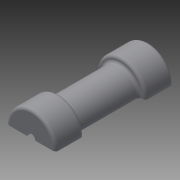
# Autodesk Inventor part: resistor
Saved by Autodesk Inventor 2015 (Build 190159000, 159)
## iProperties
Created: 2014-07-26
Part Number: resistor
Material: Generic
Document SubType Name: Modeling
Designer: dan
Density: 1 g/cm^3
Appearance: Default
Author: dan
Autodesk Inventor part; units mm, degrees
ref_plane "YZ Plane" through (0, 0, 0) normal (1, 0, 0) x (0, 1, 0)
ref_plane "XZ Plane" through (0, 0, 0) normal (0, 1, 0) x (-1, 0, 0)
ref_plane "XY Plane" through (0, 0, 0) normal (0, 0, 1) x (1, 0, 0)
sketch "Sketch1" plane through (0, 0, 0) normal (0, 1, 0) x (-1, 0, 0)
  arc A0 (379.6785, 346.6237) -> (348.5368, 347.4661) centre (364.5795, 364.4873) ccw
  circle A1 centre (364.5795, 364.4873) radius 10.6303
  line L0 (0, 0) -> (12.7, 0)
  line L1 (12.7, 0) -> (12.7, -14.605)
  line L2 (12.7, -14.605) -> (0, -14.605)
  line L3 (0, -14.605) -> (0, 0)
  line L4 (0, -14.605) -> (9.525, -14.605)
  line L5 (9.525, -14.605) -> (9.525, -46.355)
  line L6 (9.525, -46.355) -> (0, -46.355)
  line L7 (0, -46.355) -> (0, -14.605)
  line L8 (0, -46.355) -> (12.7, -46.355)
  line L9 (12.7, -46.355) -> (12.7, -60.96)
  line L10 (12.7, -60.96) -> (0, -60.96)
  line L11 (0, -60.96) -> (0, -46.355)
  point P0 (0, 0)
  dimension "d2" = 12.7
  dimension "d3" = 3.175
  dimension "d4" = 60.96
  dimension "d5" = 31.75
  constraints: 24 end point, 6 parallel, 3 horizontal, 3 perpendicular, 2 centre point, 2 equal length, 2 point on circle, 1 coincident, 1 other
  measures "d2" distance of L0.start L0.end
  measures "d3" distance between parallel lines of L5 L9
  measures "d4" distance between parallel lines of L10 L0
  measures "d5" distance of L4.end L5.end
revolve "Revolution1" add sketch "Sketch1" angle 180 about axis through (0, 0, -14.605) along (0, 0, -1) contours L0 L1 L2 L3 | L2 L5 L6 L7 | L6 L8 L9 L10 L11
sketch "Sketch2" plane through (0, 0, 0) normal (0, 0, 1) x (1, 0, 0)
  circle A0 centre (0, 0) radius 2.159
  dimension "d7" = 4.318
  constraints: 1 centre point, 1 coincident
  measures "d7" diameter of A0
extrude "Extrusion1" cut sketch "Sketch2" against normal through all
fillet "Fillet1" radius 1.5875 6 edges at (0, 12.7, 0) (0, 12.7, -14.605) (0, 12.7, -46.355) (0, 12.7, -60.96) (0, 9.525, -46.355) (0, 9.525, -14.605)
sketch "Sketch3" plane through (-2.159, 0, -60.96) normal (0, -1, 0) x (1, 0, 0)
  line L0 (4.318, 60.96) -> (4.318, 0) projected
  line L1 (0, 0) -> (0, 60.96) projected
  line L2 (7.239, 21.267) -> (-2.921, 21.267)
  line L3 (-2.921, 21.267) -> (-2.921, 39.693)
  line L4 (-2.921, 39.693) -> (7.239, 39.693)
  line L5 (7.239, 39.693) -> (7.239, 21.267)
  line L6 (2.159, 21.267) -> (2.159, 0) construction
  line L7 (4.318, 0) -> (0, 0) projected
  line L8 (11.684, 16.1925) -> (11.684, 44.7675) projected
  line L9 (11.684, 30.48) -> (7.239, 30.48)
  point P0 (2.159, 60.96)
  dimension "d11" = 10.16
  constraints: 12 end point, 4 midpoint, 2 horizontal, 2 parallel, 1 perpendicular, 1 vertical
  measures "d11" distance of L2.start L2.end
extrude "Extrusion2" cut sketch "Sketch3" against normal blind 2.54 contours L4 L5 L2 L0 | L0 L2 L1 L4 | L1 L2 L3 L4
body "Solid1"
